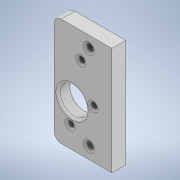
# Autodesk Inventor part: Tapa motor
Saved by Autodesk Inventor 2020 (Build 240168000, 168)
## iProperties
Created: 2020-11-22
Part Number: Tapa motor
Material: Generic
Document SubType Name: Modeling
Designer: michelin
Density: 1 g/cm^3
Appearance: Default
Author: michelin
Autodesk Inventor part; units mm, degrees
ref_plane "YZ Plane" through (0, 0, 0) normal (1, 0, 0) x (0, 1, 0)
ref_plane "XZ Plane" through (0, 0, 0) normal (0, 1, 0) x (-1, 0, 0)
ref_plane "XY Plane" through (0, 0, 0) normal (0, 0, 1) x (1, 0, 0)
sketch "Sketch1" plane through (0, 0, 0) normal (0, 0, 1) x (1, 0, 0)
  line L0 (-42.103451, 25.832396) -> (-42.103451, 67.632396)
  line L1 (-42.103451, 67.632396) -> (-67.145108, 67.632396)
  line L2 (-67.145108, 67.632396) -> (-67.145108, 20.777189)
  line L3 (-67.145108, 20.777189) -> (-42.103451, 20.777189)
  line L4 (-42.103451, 20.777189) -> (-42.103451, 67.632396)
  line L5 (-42.103451, 67.632396) -> (-64.103451, 67.632396)
  line L6 (-42.103451, 67.632396) -> (-42.103451, 62.632396)
  line L7 (-42.103451, 36.232396) -> (-42.103451, 20.832396)
  line L8 (-42.103451, 20.832396) -> (-42.103451, 25.832396)
  circle A0 centre (-52.103451, 62.632396) radius 1.5
  circle A1 centre (-52.103451, 25.832396) radius 1.5
  arc A2 (-67.103451, 26.001195) -> (-67.103451, 62.678375) centre (-65.601409, 44.339785) ccw
  circle A3 centre (-65.613731, 44.346133) radius 18.4
  circle A4 centre (-75.593787, 32.452366) radius 0.975975
  circle A5 centre (-60.312419, 29.780898) radius 1.25
  circle A6 centre (-60.312419, 29.780898) radius 1.25
  circle A7 centre (-75.593787, 32.452366) radius 0.975975
  circle A8 centre (-80.878251, 47.03768) radius 1.25
  circle A9 centre (-80.878251, 47.03768) radius 1.25
  circle A10 centre (-70.868197, 58.967198) radius 1.013606
  circle A11 centre (-50.302365, 41.710416) radius 1.254816
  circle A12 centre (-59.45554, 38.999939) radius 6.0198
  circle A13 centre (-55.614516, 56.262734) radius 1.2573
  point P0 (0, 0)
  point P1 (-62.028451, 25.832396)
  point P2 (-78.421274, 29.082698)
  constraints: 18 end point, 14 centre point, 3 coincident, 2 parallel, 2 point on circle, 1 collinear, 1 concentric, 1 horizontal, 1 perpendicular, 1 point on line
sketch "Sketch1 outline for Extrusion1" plane through (0, 0, 0) normal (0, 0, 1) x (1, 0, 0)
  line L0 (-67.145108, 67.632396) -> (-67.145108, 20.777189)
  line L1 (-42.103451, 67.632396) -> (-67.145108, 67.632396)
  line L2 (-67.145108, 20.777189) -> (-42.103451, 20.777189)
  line L3 (-42.103451, 25.832396) -> (-42.103451, 67.632396)
  line L4 (-42.103451, 20.777189) -> (-42.103451, 25.832396)
  circle A0 centre (-60.312419, 29.780898) radius 1.25
  circle A1 centre (-59.45554, 38.999939) radius 6.0198
  circle A2 centre (-52.103451, 25.832396) radius 1.5
  circle A3 centre (-50.302365, 41.710416) radius 1.254816
  circle A4 centre (-55.614516, 56.262734) radius 1.2573
  circle A5 centre (-52.103451, 62.632396) radius 1.5
extrude "Extrusion1" add sketch "Sketch1 outline for Extrusion1" against normal blind 6
fillet "Fillet1" radius 1 7 edges at (-53.6035, 62.6324, 0) (-56.8718, 56.2627, 0) (-51.5572, 41.7104, 0) (-53.6035, 25.8324, 0) (-61.5624, 29.7809, 0) (-65.4753, 38.9999, -6) (-65.4753, 38.9999, 0)
fillet "Fillet2" radius 3 2 edges at (-67.1451, 67.6324, -3) (-67.1451, 20.7772, -3)
body "Solid1"
